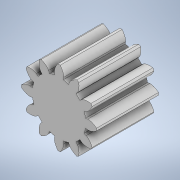
# Autodesk Inventor part: 12_Tooth_Gear
Saved by Autodesk Inventor 2021 (Build 250183000, 183)
## iProperties
Created: 2021-03-24
Part Number: 12_Tooth_Gear
Material: Generic
Document SubType Name: Modeling
Designer: lucia
Density: 1 g/cm^3
Appearance: Default
Author: lucia
Autodesk Inventor part; units mm, degrees
ref_plane "YZ Plane" through (0, 0, 0) normal (1, 0, 0) x (0, 1, 0)
ref_plane "XZ Plane" through (0, 0, 0) normal (0, 1, 0) x (-1, 0, 0)
ref_plane "XY Plane" through (0, 0, 0) normal (0, 0, 1) x (1, 0, 0)
sketch "Sketch1" plane through (0, 0, 0) normal (0, 0, 1) x (1, 0, 0)
  circle A0 centre (0, 0) radius 26.416
  dimension "d0" = 52.832
  constraints: 1 centre point, 1 coincident
  measures "d0" diameter of A0
extrude "Extrusion1" add sketch "Sketch1" against normal blind 50.8
sketch "Sketch2" plane through (0, 0, 0) normal (0, 0, 1) x (1, 0, 0)
  circle A0 centre (0, 0) radius 22.0133
  circle A1 centre (0, 0) radius 26.416
  dimension "d3" = 44.0267
  dimension "d4" = 52.832
  constraints: 2 centre point, 2 coincident
  measures "d3" diameter of A0
  measures "d4" diameter of A1
extrude "Extrusion2" cut sketch "Sketch2" against normal blind 50.8
sketch "Sketch3" plane through (0, 0, 0) normal (0, 0, 1) x (1, 0, 0)
  circle A0 centre (0, 0) radius 22.0133 projected
  circle A1 centre (0, 0) radius 23.941
  circle A2 centre (0, 0) radius 22.0133
  circle A3 centre (0, 0) radius 26.416
  circle A4 centre (0, 0) radius 30.8187
  line L0 (0, 0) -> (3.8378, 23.6314)
  line L1 (0, 0) -> (1.9552, 23.8611)
  line L2 (0, 0) -> (0.0604, 23.941)
  line L3 (0, 0) -> (-1.8348, 23.8706)
  line L4 (0, 0) -> (-3.7185, 23.6505)
  line L5 (0, 0) -> (-5.5789, 23.2819)
  line L6 (0, 0) -> (-7.4043, 22.7673)
  line L7 (0, 0) -> (-9.1832, 22.1098)
  line L8 (3.8378, 23.6314) -> (1.9552, 23.8611)
  line L9 (1.9552, 23.8611) -> (0.0604, 23.941)
  line L10 (0.0604, 23.941) -> (-1.8348, 23.8706)
  line L11 (-1.8348, 23.8706) -> (-3.7185, 23.6505)
  line L12 (-3.7185, 23.6505) -> (-5.5789, 23.2819)
  line L13 (-5.5789, 23.2819) -> (-7.4043, 22.7673)
  line L14 (-7.4043, 22.7673) -> (-9.1832, 22.1098)
  line L15 (0, 0) -> (-10.9045, 21.3135)
  line L16 (0, 0) -> (-12.5573, 20.3835)
  line L17 (-9.1832, 22.1098) -> (-10.9045, 21.3135)
  line L18 (-10.9045, 21.3135) -> (-12.5573, 20.3835)
  line L19 (1.9552, 23.8611) -> (3.8454, 23.7062)
  line L20 (0.0604, 23.941) -> (3.8535, 23.9314)
  line L21 (-3.7185, 23.6505) -> (3.7755, 24.8288)
  line L22 (-5.5789, 23.2819) -> (3.6427, 25.4917)
  line L23 (-7.4043, 22.7673) -> (3.417, 26.2866)
  line L24 (-9.1832, 22.1098) -> (3.0771, 27.202)
  line L25 (-10.9045, 21.3135) -> (2.6026, 28.224)
  line L26 (-12.5573, 20.3835) -> (1.9751, 29.3363)
  line L27 (-1.8348, 23.8706) -> (3.838, 24.3067)
  line L28 (0, 0) -> (-14.1314, 19.3256)
  line L29 (0, 0) -> (-15.6167, 18.1463)
  line L30 (-12.5573, 20.3835) -> (-14.1314, 19.3256)
  line L31 (-14.1314, 19.3256) -> (-15.6167, 18.1463)
  line L32 (-14.1314, 19.3256) -> (1.1777, 30.52)
  line L33 (-15.6167, 18.1463) -> (0.1957, 31.7546)
  spline S0 degree 4 poles (3.8378, 23.6314) (3.845, 23.6769) (3.8623, 23.9014) (3.851, 24.2798) (3.772, 24.9133) (3.6351, 25.5723) (3.406, 26.3676) (3.0621, 27.2819) (2.3775, 28.7446) (1.5854, 30.0179) (0.8213, 31.0281) (0.1957, 31.7546) knots 0 0 0 0 0 0.118311 0.18803 0.26924 0.360382 0.460423 0.568608 0.684353 1 1 1 1 1
  line L34 (0, 0) -> (0, 46.5046)
  line L35 (3.448, 26.19) -> (0, 0)
  line L36 (0, 0) -> (5.6975, 21.2632)
  arc A5 (3.8378, 23.6314) -> (5.6975, 21.2632) centre (6.3471, 23.6876) ccw
  spline S1 degree 4 poles (-3.8378, 23.6314) (-3.845, 23.6769) (-3.8623, 23.9014) (-3.851, 24.2798) (-3.772, 24.9133) (-3.6351, 25.5723) (-3.406, 26.3676) (-3.0621, 27.2819) (-2.3775, 28.7446) (-1.5854, 30.0179) (-0.8213, 31.0281) (-0.1957, 31.7546) knots 0 0 0 0 0 0.118311 0.18803 0.26924 0.360382 0.460423 0.568608 0.684353 1 1 1 1 1
  arc A6 (-5.6975, 21.2632) -> (-3.8378, 23.6314) centre (-6.3471, 23.6876) ccw
  line L37 (0, 0) -> (-3.8378, 23.6314)
  point P0 (-3.8454, 23.7062)
  point P1 (-3.8535, 23.9314)
  point P2 (-3.7755, 24.8288)
  point P3 (-3.6427, 25.4917)
  point P4 (-3.417, 26.2866)
  point P5 (-3.0771, 27.202)
  point P6 (-2.6026, 28.224)
  point P7 (-1.9751, 29.3363)
  point P8 (-3.838, 24.3067)
  point P9 (-1.1777, 30.52)
  point P10 (0.9662, 30.8035)
  point P11 (-0.9662, 30.8035)
  point P12 (-5.6975, 21.2632)
  point P13 (3.5288, 21.7287)
  point P14 (-3.5288, 21.7287)
  dimension "d8" = 52.832
  dimension "d9" = 44.0267
  dimension "d10" = 47.882
  dimension "d7" = 61.6373
  dimension "d11" = 1.8965
  dimension "d12" = 1.8965
  dimension "d13" = 3.7931
  dimension "d14" = 5.6896
  dimension "d15" = 7.5861
  dimension "d16" = 9.4827
  dimension "d17" = 11.3792
  dimension "d19" = 13.2757
  dimension "d20" = 15.1723
  dimension "d22" = 17.0688
  dimension "d23" = 18.9653
  dimension "d24" = 20.8619
  dimension "d25" = 7.5
  dimension "d26" = 15
  constraints: 76 end point, 14 symmetric about line, 10 equal length, 4 coincident, 4 point on circle, 3 centre point, 1 tangent, 1 vertical, 57 other
  measures "d7" diameter of A4
  measures "d11" distance of L0.end L1.end
  measures "d12" distance of L1.end L19.end
  measures "d13" distance of L2.end L20.end
  measures "d14" distance of L3.end L27.end
  measures "d15" distance of L4.end L21.end
  measures "d16" distance of L5.end L22.end
  measures "d17" distance of L6.end L23.end
  measures "d19" distance of L7.end L24.end
  measures "d20" distance of L15.end L25.end
  measures "d22" distance of L16.end L26.end
  measures "d23" distance of L28.end L32.end
  measures "d24" distance of L29.end L33.end
  measures "d25" angle of L34 L35
  measures "d26" angle of L34 L36
extrude "Extrusion3" add sketch "Sketch3" against normal blind 50.8 contours A0 L35 L8 L0 | L8 L35 A1 | A1 L35 L19 S0 | A0 L1 L8 L35 | A0 L2 L9 L1 | A0 L34 A1 L2 | L3 L10 L34 A0 | A0 L4 L11 L3 | A0 L37 L12 L4 | L35 L8 A1 | A1 L19 L35 | L19 L35 L20 S0 | L9 A1 | A1 L20 L35 L19 | A1 L34 L27 L35 L20 | L11 A1 | L27 L34 A1 | A1 L10 | A1 L21 L34 L27 | L12 A6 A1 | A1 S1 L22 L34 L21 | L20 L35 L27 S0 | S1 A4 L33 | L33 A4 L34 L32 S1 | L34 L21 L35 L27 | L34 L22 L35 L21 | S1 L24 L34 L23 | L23 L34 L22 S1 | S1 L25 A3 L34 L24 | S1 L26 A3 L25 | S1 A3 L26 | L27 L35 L21 S0 | S1 L32 L34 L26 A3 | L35 L22 L34 L23 A3 | A3 L23 S0 | S0 L22 L35 | L35 L22 S0 L21 | L34 L24 A3 L23 | L34 A3 L24 | L25 L34 A3 | A3 L26 L34 L25 | L34 A4 S0 L32 | L32 S0 L26 L34 | A3 L24 S0 L23 | A3 L34 L25 S0 L24 | L34 L26 S0 L25 picked at (-3.7716, 23.6405)
pattern_circular "Circular Pattern1" count 12 over 360 about axis through (0, 0, 0) along (0, 0, -1) of "Extrusion3"
equation "\"d0\" = 13.208 * scale"
equation "\"d1\" = 12.7 * scale"
equation "\"d3\" = 11.0067 * scale"
equation "\"d4\" = 13.208 * scale"
equation "\"d5\" = 12.7 * scale"
equation "\"d8\" = 13.208 * scale"
equation "\"d9\" = 11.0067 * scale"
equation "\"d10\" = 11.9705 * scale"
equation "\"d7\" = 15.4093 * scale"
equation "\"d27\" = 12.7 * scale"
equation "\"prcsn\" = 0.47413"
equation "\"scale\" = 4"
body "Solid1"
